# Autodesk Inventor part: Board
Saved by Autodesk Inventor 2021 (Build 250183000, 183)
## iProperties
Created: 2021-01-20
Part Number: Board
Material: Generic
Document SubType Name: Modeling
Designer: User
Density: 1 g/cm^3
Appearance: Default
Author: User
Autodesk Inventor part; units mm, degrees
ref_plane "YZ Plane" through (0, 0, 0) normal (1, 0, 0) x (0, 1, 0)
ref_plane "XZ Plane" through (0, 0, 0) normal (0, 1, 0) x (-1, 0, 0)
ref_plane "XY Plane" through (0, 0, 0) normal (0, 0, 1) x (1, 0, 0)
sketch "board" plane through (0, 0, 0) normal (0, 0, 1) x (1, 0, 0)
  line L0 (22.5, 10) -> (-22.5, 10)
  line L1 (-22.5, 10) -> (-22.5, -10)
  line L2 (-22.5, -10) -> (22.5, -10)
  line L3 (22.5, -10) -> (22.5, 10)
  line L4 (22.5, 10) -> (-22.5, -10) construction
  line L5 (-22.5, 10) -> (22.5, -10) construction
  circle A0 centre (-3.81, -8) radius 0.5
  circle A1 centre (-21.25, 8.75) radius 0.8
  circle A2 centre (21.25, 8.75) radius 0.8
  circle A3 centre (-21.25, -8.75) radius 0.8
  circle A4 centre (21.25, -8.75) radius 0.8
  circle A5 centre (-1.27, -8) radius 0.5
  circle A6 centre (1.27, -8) radius 0.5
  circle A7 centre (3.81, -8) radius 0.5
  circle A8 centre (-2.44, 7) radius 0.5
  circle A9 centre (2.44, 7) radius 0.5
  circle A10 centre (-13.1, 5.1) radius 0.75
  circle A11 centre (13.1, 5.1) radius 0.75
  circle A12 centre (-13.1, -5.1) radius 0.75
  circle A13 centre (13.1, -5.1) radius 0.75
  point P0 (0, 0)
  point P1 (0, 0)
  point P2 (13.2529, 5)
  dimension "d34" = 45
  dimension "d35" = 20
  dimension "d39" = 1
  dimension "d44" = 1.6
  dimension "d48" = 1.25
  dimension "d51" = 42.5
  dimension "d54" = 17.5
  dimension "d57" = 1.25
  dimension "d60" = 2.54
  dimension "d65" = 3.81
  dimension "d66" = 2
  dimension "d67" = 4.88
  dimension "d68" = 2.44
  dimension "d69" = 1
  dimension "d70" = 1
  dimension "d71" = 3
  dimension "d72" = 1.5
  dimension "d75" = 26.2
  dimension "d78" = 10.2
  dimension "d81" = 5.1
  dimension "d82" = 13.1
  constraints: 14 centre point, 12 end point, 4 horizontal, 2 midpoint, 2 parallel, 2 vertical, 1 coincident, 1 horizontal alignment, 1 perpendicular, 18 other
  measures "d34" distance of L1.end L2.end
  measures "d35" distance of L2.end L0.start
  measures "d39" diameter of A0
  measures "d44" diameter of A1
  measures "d48" distance from line of L0 A1.centre
  measures "d51" distance of A1.centre A2.centre
  measures "d54" distance of A1.centre A3.centre
  measures "d57" distance from line of L1 A1.centre
  measures "d60" distance of A0.centre A5.centre
  measures "d65" horizontal distance of point (0, 0) A0.centre
  measures "d66" distance from line of L2 A0.centre
  measures "d67" distance of A9.centre A8.centre
  measures "d68" horizontal distance of point (0, 0) A8.centre
  measures "d69" diameter of A8
  measures "d70" diameter of A9
  measures "d71" distance from line of L0 A8.centre
  measures "d72" diameter of A10
  measures "d75" distance of A10.centre A11.centre
  measures "d78" distance of A10.centre A12.centre
  measures "d81" vertical distance of point (0, 0) A10.centre
  measures "d82" horizontal distance of point (0, 0) A10.centre
extrude "Extrusion2" add sketch "board" along normal blind 1.5
equation "\"d68\" = 0.5 * d67"
equation "\"d70\" = d69"
equation "\"d81\" = 0.5 * d78"
equation "\"d82\" = 0.5 * d75"
body "Solid2"
